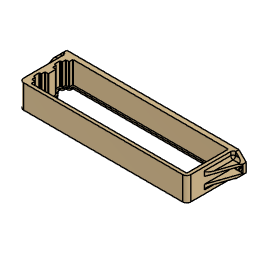
Porta Fusivel v7 (Autodesk Fusion 360 design; units mm, degrees)
Autodesk Fusion 360 part; units mm, degrees
sketch "Sketch1" plane through (0, 0, 0) normal (0, 0, 1) x (1, 0, 0)
  line L0 (0, 0) -> (197, 0)
  line L1 (197, 0) -> (197, 25.5)
  line L2 (195.5, 25.5) -> (0, 25.5)
  line L3 (0, 25.5) -> (0, 0)
  line L4 (6.5, 25.5) -> (6.5, 20.8)
  line L5 (6.5, 20.8) -> (2.5, 20.8)
  line L6 (0, 12.75) -> (197, 12.75) construction
  line L7 (197, 17.5) -> (188, 17.5)
  line L8 (188, 17.5) -> (188, 8)
  line L9 (188, 8) -> (197, 8)
  line L10 (6.5, 4.7) -> (2.5, 4.7)
  line L11 (6.5, 0) -> (6.5, 4.7)
  line L12 (2.5, 20.8) -> (2.5, 16.25)
  line L13 (2.5, 16.25) -> (0, 16.25)
  line L14 (2.5, 4.7) -> (2.5, 9.25)
  line L15 (2.5, 9.25) -> (0, 9.25)
  line L16 (0, 25.5) -> (0, 51)
  line L17 (0, 51) -> (197, 51)
  line L18 (6.5, 46.3) -> (2.5, 46.3)
  line L19 (6.5, 51) -> (6.5, 46.3)
  line L20 (2.5, 41.75) -> (0, 41.75)
  line L21 (2.5, 46.3) -> (2.5, 41.75)
  line L22 (6.5, 25.5) -> (6.5, 30.2)
  line L23 (6.5, 30.2) -> (2.5, 30.2)
  line L24 (2.5, 30.2) -> (2.5, 34.75)
  line L25 (2.5, 34.75) -> (0, 34.75)
  line L26 (197, 33.5) -> (188, 33.5)
  line L27 (188, 33.5) -> (188, 43)
  line L28 (188, 43) -> (197, 43)
  line L29 (197, 51) -> (197, 25.5)
  line L30 (201, -4) -> (201, 25.5)
  line L31 (201, 55) -> (201, 25.5)
  line L32 (-4, 55) -> (201, 55)
  line L33 (-4, 25.5) -> (-4, 55)
  line L34 (-4, 25.5) -> (-4, -4)
  line L35 (-4, -4) -> (201, -4)
  point P0 (0, 25.5)
  dimension "d1" = 25.5
  dimension "d2" = 197
  dimension "d5" = 4.7
  dimension "d6" = 4
  dimension "d7" = 9
  dimension "d8" = 9.5
  dimension "d9" = 2.5
  dimension "d10" = 7
  dimension "d19" = 4
  constraint horizontal L0
  constraint vertical L1
  constraint horizontal L2
  constraint vertical L3
  constraint coincident L0.start L3.end
  constraint coincident P0 L2
  constraint coincident P0 L3
  constraint coincident L3.end L0
  constraint coincident L0.start L3
  constraint coincident L2 L4.start
  constraint perpendicular L2 L4
  constraint perpendicular L3 L5
  constraint midpoint L3 L6.start
  constraint perpendicular L3 L6
  constraint midpoint L1 L6.end
  constraint coincident L1 L7.start
  constraint perpendicular L1 L7
  constraint perpendicular L6 L8
  constraint coincident L1 L9.end
  constraint perpendicular L1 L9
  constraint symmetric L6 L7 L9
  constraint symmetric L4.start L6 L11.start
  constraint symmetric L4.end L6 L10.start
  constraint symmetric L5.end L6 L10.end
  constraint perpendicular L5 L12
  constraint coincident L3 L13.end
  constraint perpendicular L3 L13
  constraint symmetric L6 L12.end L14.end
  constraint symmetric L6 L13.end L15.end
  constraint coincident P0 L2.end
  constraint coincident L0.end L1.start
  constraint symmetric L2 P0 L3.start
  constraint symmetric L2 L1.end L29.end
  constraint symmetric L2 L0.end L17.end
  constraint symmetric L2 L0.start L16.end
  constraint symmetric L2 L4.start L22.start
  constraint symmetric L2 L4.end L22.end
  constraint symmetric L2 L5.end L23.end
  constraint symmetric L2 L7.start L26.start
  constraint symmetric L2 L7.end L26.end
  constraint symmetric L2 L8.end L27.end
  constraint symmetric L2 L9.end L28.end
  constraint symmetric L2 L10.start L18.start
  constraint symmetric L2 L10.end L18.end
  constraint symmetric L2 L11.start L19.start
  constraint symmetric L2 L12.end L24.end
  constraint symmetric L2 L13.end L25.end
  constraint symmetric L2 L14.end L20.start
  constraint symmetric L2 L15.end L20.end
  measures "d1" distance of L0.start P0
  measures "d2" distance of L1 L3
  measures "d5" distance of L4.start L4.end
  measures "d6" distance of L4.end L5.end
  measures "d7" distance of L7.start L7.end
  measures "d8" distance of L7.end L8.end
  measures "d9" distance of L12.end L13.end
  measures "d10" distance of L13 L15
extrude "Extrude1" add sketch "Sketch1" against normal blind 2 contours L0 L3 L10 L11 L14 L15 | L2 L3 L4 L5 L12 L13 | L1 L7 L8 L9 | L2 L16 L22 L23 L24 L25 | L16 L17 L18 L19 L20 L21 | L26 L27 L28 L29 | L30 L31 L32 L33 L34 L35
extrude "Extrude2" add sketch "Sketch1" along normal blind 9 contours L1 L7 L8 L9 | L26 L27 L28 L29
extrude "Extrude3" add sketch "Sketch1" along normal blind 27 contours L0 L3 L10 L11 L14 L15 | L2 L3 L4 L5 L12 L13 | L2 L16 L22 L23 L24 L25 | L16 L17 L18 L19 L20 L21 | L30 L31 L32 L33 L34 L35
fillet "Fillet1" radius 0.5 26 edges at (6.5, 20.8, 12.5) (2.5, 20.8, 12.5) (2.5, 16.25, 12.5) (0, 16.25, 12.5) (2.5, 9.25, 12.5) (2.5, 4.7, 12.5) (6.5, 4.7, 12.5) (6.5, 0, 12.5) (6.5, 30.2, 12.5) (2.5, 34.75, 12.5) (2.5, 30.2, 12.5) (6.5, 46.3, 12.5) (2.5, 46.3, 12.5) (2.5, 41.75, 12.5) (6.5, 51, 12.5) (0, 41.75, 12.5) (0, 34.75, 12.5) (0, 9.25, 12.5) (188, 43, 3.5) (188, 33.5, 3.5) (188, 17.5, 3.5) (188, 8, 3.5) (197, 33.5, 3.5) (197, 43, 3.5) (197, 17.5, 3.5) (197, 8, 3.5)
fillet "Fillet2" radius 1 2 edges at (197, 51, 12.5) (197, 0, 12.5)
fillet "Fillet3" radius 5 2 edges at (201, -4, 12.5) (-4, -4, 12.5)
sketch "Sketch3" plane through (0, 0, -2) normal (0, 0, -1) x (1, 0, 0)
  arc A0 (1, 4) -> (-4, -1) centre (1, -1) ccw
  line L0 (-4, -1) -> (-4, -55)
  line L1 (-4, -55) -> (201, -55)
  line L2 (201, -55) -> (201, -1)
  arc A1 (201, -1) -> (196, 4) centre (196, -1) ccw
  line L3 (196, 4) -> (1, 4)
  arc A2 (188.5, -8) -> (188, -8.5) centre (188.5, -8.5) ccw
  line L4 (188, -8.5) -> (188, -17)
  arc A3 (188, -17) -> (188.5, -17.5) centre (188.5, -17) ccw
  line L5 (188.5, -17.5) -> (196.5, -17.5)
  arc A4 (197, -18) -> (196.5, -17.5) centre (196.5, -18) ccw
  line L6 (197, -18) -> (197, -33)
  arc A5 (196.5, -33.5) -> (197, -33) centre (196.5, -33) ccw
  line L7 (196.5, -33.5) -> (188.5, -33.5)
  arc A6 (188.5, -33.5) -> (188, -34) centre (188.5, -34) ccw
  line L8 (188, -34) -> (188, -42.5)
  arc A7 (188, -42.5) -> (188.5, -43) centre (188.5, -42.5) ccw
  line L9 (188.5, -43) -> (196.5, -43)
  arc A8 (197, -43.5) -> (196.5, -43) centre (196.5, -43.5) ccw
  line L10 (197, -43.5) -> (197, -50)
  arc A9 (196, -51) -> (197, -50) centre (196, -50) ccw
  line L11 (196, -51) -> (7, -51)
  arc A10 (6.5, -50.5) -> (7, -51) centre (7, -50.5) ccw
  line L12 (6.5, -50.5) -> (6.5, -46.8)
  arc A11 (6.5, -46.8) -> (6, -46.3) centre (6, -46.8) ccw
  line L13 (6, -46.3) -> (3, -46.3)
  arc A12 (2.5, -45.8) -> (3, -46.3) centre (3, -45.8) ccw
  line L14 (2.5, -45.8) -> (2.5, -42.25)
  arc A13 (2.5, -42.25) -> (2, -41.75) centre (2, -42.25) ccw
  line L15 (2, -41.75) -> (0.5, -41.75)
  arc A14 (0, -41.25) -> (0.5, -41.75) centre (0.5, -41.25) ccw
  line L16 (0, -41.25) -> (0, -35.25)
  arc A15 (0.5, -34.75) -> (0, -35.25) centre (0.5, -35.25) ccw
  line L17 (0.5, -34.75) -> (2, -34.75)
  arc A16 (2, -34.75) -> (2.5, -34.25) centre (2, -34.25) ccw
  line L18 (2.5, -34.25) -> (2.5, -30.7)
  arc A17 (3, -30.2) -> (2.5, -30.7) centre (3, -30.7) ccw
  line L19 (3, -30.2) -> (6, -30.2)
  arc A18 (6, -30.2) -> (6.5, -29.7) centre (6, -29.7) ccw
  line L20 (6.5, -29.7) -> (6.5, -21.3)
  arc A19 (6.5, -21.3) -> (6, -20.8) centre (6, -21.3) ccw
  line L21 (6, -20.8) -> (3, -20.8)
  arc A20 (2.5, -20.3) -> (3, -20.8) centre (3, -20.3) ccw
  line L22 (2.5, -20.3) -> (2.5, -16.75)
  arc A21 (2.5, -16.75) -> (2, -16.25) centre (2, -16.75) ccw
  line L23 (2, -16.25) -> (0.5, -16.25)
  arc A22 (0, -15.75) -> (0.5, -16.25) centre (0.5, -15.75) ccw
  line L24 (0, -15.75) -> (0, -9.75)
  arc A23 (0.5, -9.25) -> (0, -9.75) centre (0.5, -9.75) ccw
  line L25 (0.5, -9.25) -> (2, -9.25)
  arc A24 (2, -9.25) -> (2.5, -8.75) centre (2, -8.75) ccw
  line L26 (2.5, -8.75) -> (2.5, -5.2)
  arc A25 (3, -4.7) -> (2.5, -5.2) centre (3, -5.2) ccw
  line L27 (3, -4.7) -> (6, -4.7)
  arc A26 (6, -4.7) -> (6.5, -4.2) centre (6, -4.2) ccw
  line L28 (6.5, -4.2) -> (6.5, -0.5)
  arc A27 (7, 0) -> (6.5, -0.5) centre (7, -0.5) ccw
  line L29 (7, 0) -> (196, 0)
  arc A28 (197, -1) -> (196, 0) centre (196, -1) ccw
  line L30 (197, -1) -> (197, -7.5)
  arc A29 (196.5, -8) -> (197, -7.5) centre (196.5, -7.5) ccw
  line L31 (196.5, -8) -> (188.5, -8)
  line L32 (188.5, -45) -> (195, -45)
  line L33 (195, -45) -> (195, -49)
  line L34 (195, -49) -> (8.5, -49)
  line L35 (8.5, -49) -> (8.5, -46.8)
  arc A30 (8.5, -46.8) -> (6, -44.3) centre (6, -46.8) ccw
  line L36 (6, -44.3) -> (4.5, -44.3)
  line L37 (4.5, -44.3) -> (4.5, -42.25)
  arc A31 (4.5, -42.25) -> (2, -39.75) centre (2, -42.25) ccw
  line L38 (2, -39.75) -> (2, -36.75)
  arc A32 (2, -36.75) -> (4.5, -34.25) centre (2, -34.25) ccw
  line L39 (4.5, -34.25) -> (4.5, -32.2)
  line L40 (4.5, -32.2) -> (6, -32.2)
  arc A33 (6, -32.2) -> (8.5, -29.7) centre (6, -29.7) ccw
  line L41 (8.5, -29.7) -> (8.5, -21.3)
  arc A34 (8.5, -21.3) -> (6, -18.8) centre (6, -21.3) ccw
  line L42 (6, -18.8) -> (4.5, -18.8)
  line L43 (4.5, -18.8) -> (4.5, -16.75)
  arc A35 (4.5, -16.75) -> (2, -14.25) centre (2, -16.75) ccw
  line L44 (2, -14.25) -> (2, -11.25)
  arc A36 (2, -11.25) -> (4.5, -8.75) centre (2, -8.75) ccw
  line L45 (4.5, -8.75) -> (4.5, -6.7)
  line L46 (4.5, -6.7) -> (6, -6.7)
  arc A37 (6, -6.7) -> (8.5, -4.2) centre (6, -4.2) ccw
  line L47 (8.5, -4.2) -> (8.5, -2)
  line L48 (8.5, -2) -> (195, -2)
  line L49 (195, -2) -> (195, -6)
  line L50 (195, -6) -> (188.5, -6)
  arc A38 (188.5, -6) -> (186, -8.5) centre (188.5, -8.5) ccw
  line L51 (186, -8.5) -> (186, -17)
  arc A39 (186, -17) -> (188.5, -19.5) centre (188.5, -17) ccw
  line L52 (188.5, -19.5) -> (195, -19.5)
  line L53 (195, -19.5) -> (195, -31.5)
  line L54 (195, -31.5) -> (188.5, -31.5)
  arc A40 (188.5, -31.5) -> (186, -34) centre (188.5, -34) ccw
  line L55 (186, -34) -> (186, -42.5)
  arc A41 (186, -42.5) -> (188.5, -45) centre (188.5, -42.5) ccw
  dimension "d24" = 2
extrude "Extrude4" add sketch "Sketch3" against normal blind 2 contours A2 L4 A3 L5 A4 L6 A5 L7 A6 L8 A7 L9 A8 L10 A9 L11 A10 L12 A11 L13 A12 L14 A13 L15 A14 L16 A15 L17 A16 L18 A17 L19 A18 L20 A19 L21 A20 L22 A21 L23 A22 L24 A23 L25 A24 L26 A25 L27 A26 L28 A27 L29 A28 L30 A29 L31
sketch "Sketch4" plane through (0, 0, 27) normal (0, 0, 1) x (-1, 0, 0)
  arc A0 (-2, -41.75) -> (-2.5, -42.25) centre (-2, -42.25) ccw
  line L0 (-2.5, -42.25) -> (-2.5, -45.8)
  arc A1 (-3, -46.3) -> (-2.5, -45.8) centre (-3, -45.8) ccw
  line L1 (-3, -46.3) -> (-6, -46.3)
  arc A2 (-6, -46.3) -> (-6.5, -46.8) centre (-6, -46.8) ccw
  line L2 (-6.5, -46.8) -> (-6.5, -50.5)
  arc A3 (-7, -51) -> (-6.5, -50.5) centre (-7, -50.5) ccw
  line L3 (-7, -51) -> (-196, -51)
  arc A4 (-197, -50) -> (-196, -51) centre (-196, -50) ccw
  line L4 (-197, -50) -> (-197, -1)
  arc A5 (-196, 0) -> (-197, -1) centre (-196, -1) ccw
  line L5 (-196, 0) -> (-7, 0)
  arc A6 (-6.5, -0.5) -> (-7, 0) centre (-7, -0.5) ccw
  line L6 (-6.5, -0.5) -> (-6.5, -4.2)
  arc A7 (-6.5, -4.2) -> (-6, -4.7) centre (-6, -4.2) ccw
  line L7 (-6, -4.7) -> (-3, -4.7)
  arc A8 (-2.5, -5.2) -> (-3, -4.7) centre (-3, -5.2) ccw
  line L8 (-2.5, -5.2) -> (-2.5, -8.75)
  arc A9 (-2.5, -8.75) -> (-2, -9.25) centre (-2, -8.75) ccw
  line L9 (-2, -9.25) -> (-0.5, -9.25)
  arc A10 (0, -9.75) -> (-0.5, -9.25) centre (-0.5, -9.75) ccw
  line L10 (0, -9.75) -> (0, -15.75)
  arc A11 (-0.5, -16.25) -> (0, -15.75) centre (-0.5, -15.75) ccw
  line L11 (-0.5, -16.25) -> (-2, -16.25)
  arc A12 (-2, -16.25) -> (-2.5, -16.75) centre (-2, -16.75) ccw
  line L12 (-2.5, -16.75) -> (-2.5, -20.3)
  arc A13 (-3, -20.8) -> (-2.5, -20.3) centre (-3, -20.3) ccw
  line L13 (-3, -20.8) -> (-6, -20.8)
  arc A14 (-6, -20.8) -> (-6.5, -21.3) centre (-6, -21.3) ccw
  line L14 (-6.5, -21.3) -> (-6.5, -29.7)
  arc A15 (-6.5, -29.7) -> (-6, -30.2) centre (-6, -29.7) ccw
  line L15 (-6, -30.2) -> (-3, -30.2)
  arc A16 (-2.5, -30.7) -> (-3, -30.2) centre (-3, -30.7) ccw
  line L16 (-2.5, -30.7) -> (-2.5, -34.25)
  arc A17 (-2.5, -34.25) -> (-2, -34.75) centre (-2, -34.25) ccw
  line L17 (-2, -34.75) -> (-0.5, -34.75)
  arc A18 (0, -35.25) -> (-0.5, -34.75) centre (-0.5, -35.25) ccw
  line L18 (0, -35.25) -> (0, -41.25)
  arc A19 (-0.5, -41.75) -> (0, -41.25) centre (-0.5, -41.25) ccw
  line L19 (-0.5, -41.75) -> (-2, -41.75)
  arc A20 (4, -1) -> (-1, 4) centre (-1, -1) ccw
  line L20 (-1, 4) -> (-196, 4)
  arc A21 (-196, 4) -> (-201, -1) centre (-196, -1) ccw
  line L21 (-201, -1) -> (-201, -55)
  line L22 (-201, -55) -> (4, -55)
  line L23 (4, -55) -> (4, -1)
  line L24 (-7, -51) -> (4, -51)
  line L25 (-196, -51) -> (-201, -51)
  constraint coincident A3.start L3.start
  constraint coincident L23 L24.end
  constraint tangent A3 L24
  constraint coincident L3.end A4.end
  constraint coincident L21 L25.end
  constraint tangent A4 L25
extrude "Extrude8" add 1 faces at (64.3333, 55, 7.6667) along direction (0, 1, 0) blind 2
sketch "Sketch6" plane through (0, 57, 0) normal (0, 1, 0) x (-1, 0, 0)
  line L0 (-201, 27) -> (-201, -2)
  line L1 (-201, -2) -> (4, -2)
  line L2 (4, -2) -> (4, 27)
  line L3 (4, 27) -> (-201, 27)
  line L4 (4, 27) -> (7, 27)
  line L5 (7, 27) -> (16, 18)
  line L6 (16, 18) -> (16, 14.25)
  line L7 (16, 14.25) -> (10, 14.25)
  arc A0 (10, 14.25) -> (10, 10.75) centre (10, 12.5) ccw
  line L8 (10, 12.5) -> (4, 12.5) construction
  line L9 (4, -2) -> (7, -2)
  line L10 (7, -2) -> (16, 7)
  line L11 (16, 7) -> (16, 10.75)
  line L12 (16, 10.75) -> (10, 10.75)
  line L13 (-98.5, 27) -> (-98.5, 53.5133) construction
  line L14 (-201, 27) -> (-204, 27)
  line L15 (-213, 18) -> (-213, 14.25)
  line L16 (-213, 14.25) -> (-207, 14.25)
  arc A1 (-207, 10.75) -> (-207, 14.25) centre (-207, 12.5) ccw
  line L17 (-204, 27) -> (-213, 18)
  line L18 (-201, -2) -> (-204, -2)
  line L19 (-204, -2) -> (-213, 7)
  line L20 (-213, 7) -> (-213, 10.75)
  line L21 (-213, 10.75) -> (-207, 10.75)
  line L22 (-213, 14.25) -> (-213, 10.75)
  arc A2 (-208, 14.25) -> (-208, 10.75) centre (-208, 12.5) ccw
  arc A3 (11, 10.75) -> (11, 14.25) centre (11, 12.5) ccw
  line L23 (16, 14.25) -> (16, 10.75)
  line L24 (16, 18) -> (4, 18)
  dimension "d41" = 6
  dimension "d43" = 3.5
  dimension "d44" = 3
  dimension "d45" = 135
  dimension "d46" = 12
  dimension "d50" = 1
  constraint coincident L2.end L3.start
  constraint perpendicular L2 L4
  constraint perpendicular L4 L6
  constraint perpendicular L6 L7
  constraint tangent L7 A0
  constraint coincident A0.centre L8.start
  constraint midpoint L2 L8.end
  constraint horizontal L8
  constraint symmetric L2.end L8 L1.end
  constraint symmetric L4.end L8 L9.end
  constraint symmetric L5.end L8 L10.end
  constraint symmetric L6.end L8 L11.end
  constraint symmetric L7.end L8 A0.end
  constraint coincident A0.end L12.end
  constraint midpoint L3 L13.start
  constraint perpendicular L3 L13
  constraint symmetric L2.end L13 L0.start
  constraint symmetric L4.end L13 L14.end
  constraint symmetric L5.end L13 L15.start
  constraint symmetric L6.end L13 L15.end
  constraint symmetric L7.end L13 L16.end
  constraint symmetric A0.end L13 A1.start
  constraint symmetric A0 L13 A1
  constraint symmetric L1.end L13 L0.end
  constraint symmetric L9.end L13 L18.end
  constraint symmetric L10.end L13 L19.end
  constraint symmetric L11.end L13 L20.end
  constraint tangent L21 A2
  constraint coincident L21 A2.end
  constraint coincident L16 A2.start
  constraint tangent L16 A2
  constraint symmetric L13 A2.start A3.end
  constraint symmetric L13 A2.end A3.start
  constraint symmetric L13 A2 A3
  constraint coincident L2 L24.end
  constraint perpendicular L2 L24
  measures "d41" distance of A0.centre L8.end
  measures "d43" distance of L7.end A0.end
  measures "d44" distance of L2.end L4.end
  measures "d45" angle of L5 L6
  measures "d46" distance of L2 L6
  measures "d50" distance of A1.centre A2.centre
extrude "Extrude9" add sketch "Sketch6" against normal blind 4 contours L0 L14 L15 L16 A1 L17 L18 L19 L20 L21 | L2 L4 L5 L24 | L2 L6 L7 A0 L9 L10 L11 L12 L24 | L16 L21 L22 A2 | L7 L12 A3 L23
chamfer "Chamfer2" distance 2.2 angle 45 8 edges at (-10.5, 53, 14.25) (-8.25, 53, 12.5) (-10.5, 53, 10.75) (-12.75, 53, 12.5) (209.75, 53, 12.5) (207.5, 53, 10.75) (205.25, 53, 12.5) (207.5, 53, 14.25)
sketch "Sketch8" plane through (0, 53, 0) normal (0, -1, 0) x (1, 0, 0)
  line L0 (-7, -2) -> (-4, -2)
  line L1 (-4, -2) -> (-4, 27)
  line L2 (-4, 27) -> (-7, 27)
  line L3 (-7, 27) -> (-16, 18)
  line L4 (-16, 18) -> (-16, 7)
  line L5 (-16, 7) -> (-7, -2)
  line L6 (-11, 16.45) -> (-10, 16.45)
  arc A0 (-10, 8.55) -> (-10, 16.45) centre (-10, 12.5) ccw
  line L7 (-10, 8.55) -> (-11, 8.55)
  arc A1 (-11, 16.45) -> (-11, 8.55) centre (-11, 12.5) ccw
  line L8 (-16, 16.65) -> (-4, 16.65)
  line L9 (-14.35, 19.65) -> (-4, 19.65)
  line L10 (-16, 8.35) -> (-4, 8.35)
  line L11 (-14.35, 5.35) -> (-4, 5.35)
  line L12 (-4, 27) -> (201, 27)
  line L13 (204, 27) -> (201, 27)
  line L14 (201, 27) -> (201, -2)
  line L15 (201, -2) -> (204, -2)
  line L16 (204, -2) -> (213, 7)
  line L17 (213, 7) -> (213, 18)
  line L18 (213, 18) -> (204, 27)
  arc A2 (208, 8.55) -> (208, 16.45) centre (208, 12.5) ccw
  line L19 (208, 8.55) -> (207, 8.55)
  arc A3 (207, 16.45) -> (207, 8.55) centre (207, 12.5) ccw
  line L20 (207, 16.45) -> (208, 16.45)
  line L21 (98.5, 27) -> (98.5, 42.1012) construction
  line L22 (211.35, 19.65) -> (201, 19.65)
  line L23 (213, 16.65) -> (201, 16.65)
  line L24 (213, 8.35) -> (201, 8.35)
  line L25 (211.35, 5.35) -> (201, 5.35)
  point P0 (201, 27)
  dimension "d60" = 3
  dimension "d61" = 0.2
  dimension "d71" = 3
  constraint coincident L4 L8.start
  constraint coincident L1 L8.end
  constraint perpendicular L1 L8
  constraint coincident L3 L9.start
  constraint coincident L1 L9.end
  constraint perpendicular L1 L9
  constraint coincident L4 L10.start
  constraint coincident L1 L10.end
  constraint perpendicular L1 L10
  constraint coincident L1 L11.end
  constraint perpendicular L1 L11
  constraint coincident L5 L11.start
  constraint equal L9 L11
  constraint coincident L1.end L2.start
  constraint coincident P0 L12.end
  constraint midpoint L12 L21.start
  constraint perpendicular L12 L21
  constraint symmetric L8.start L21 L23.start
  constraint symmetric L8.end L21 L23.end
  constraint symmetric L9.start L21 L22.start
  constraint symmetric L9.end L21 L22.end
  constraint symmetric L10.start L21 L24.start
  constraint symmetric L10.end L21 L24.end
  constraint symmetric L11.start L21 L25.start
  constraint symmetric L11.end L21 L25.end
  measures "d60" distance of L8 L9
  measures "d61" distance of L6 L8
  measures "d71" distance of L10 L11
extrude "Extrude12" add sketch "Sketch8" along normal blind 0.2 contours L1 L4 L5 L10 L11 | L1 L3 L4 L8 L9 | L14 L17 L18 L22 L23 | L14 L16 L17 L24 L25
chamfer "Chamfer3" distance 35 distance2 12 4 edges at (-4, 52.8, 18.15) (-4, 52.8, 6.85) (201, 52.8, 18.15) (201, 52.8, 6.85) measured on face at (-4, 18.2667, 13.8833) measured on face at (-4, 18.2667, 13.8833) measured on face at (201, 18.2667, 11.1167) measured on face at (201, 18.2667, 11.1167)
fillet "Fillet5" radius 3 12 edges at (-9.175, 53, 19.65) (-4, 35.4, 19.65) (-4, 53, 23.325) (-4, 53, 1.675) (-9.175, 53, 5.35) (-4, 35.4, 5.35) (206.175, 53, 19.65) (201, 53, 23.325) (201, 35.4, 19.65) (201, 35.4, 5.35) (206.175, 53, 5.35) (201, 53, 1.675)
ref_plane "WorkPlane3" through (98.5, 29, 12.5) normal (-1, 0, 0) x (0, 1, 0)
equation "d2 = 94.5 mm + 94.5 mm + 4 mm + 4 mm"
